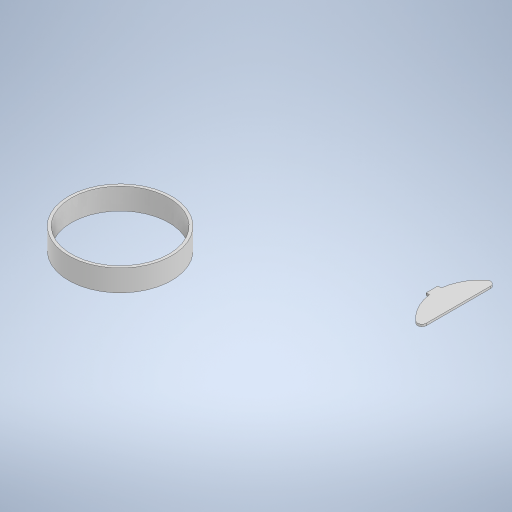
# Autodesk Inventor part: Socle test mesure
Saved by Autodesk Inventor 2024 (Build 280153000, 153)
## iProperties
Created: 2025-01-19
Part Number: Socle test mesure
Material: Générique
Document SubType Name: Modeling
Designer: malam
Density: 1 g/cm^3
Appearance: Par défaut
Author: malam
Autodesk Inventor part; units mm, degrees
ref_plane "YZ Plane" through (0, 0, 0) normal (1, 0, 0) x (0, 1, 0)
ref_plane "XZ Plane" through (0, 0, 0) normal (0, 1, 0) x (-1, 0, 0)
ref_plane "XY Plane" through (0, 0, 0) normal (0, 0, 1) x (1, 0, 0)
sketch "Esquisse1" plane through (0, 0, 0) normal (0, 1, 0) x (-1, 0, 0)
  circle A0 centre (0, 0) radius 45.31
  circle A1 centre (0, 0) radius 47.89
  arc A2 (26.876, -173.3076) -> (26.876, -102.0616) centre (-1.124, -137.6846) ccw
  line L0 (26.876, -105.1346) -> (26.876, -170.2346)
  arc A3 (26.876, -176.5363) -> (26.876, -98.8329) centre (-1.124, -137.6846) ccw
  line L1 (26.876, -170.2346) -> (26.876, -176.5363)
  line L2 (26.876, -105.1346) -> (26.876, -98.8329)
  line L3 (19.5, -32.55) -> (1.5, -32.55)
  line L4 (1.5, -32.55) -> (1.5, 32.55)
  line L5 (1.5, 32.55) -> (19.5, 32.55)
  line L6 (19.5, 32.55) -> (19.5, -32.55)
  line L7 (-1.5, -32.55) -> (-19.5, -32.55)
  line L8 (-19.5, -32.55) -> (-19.5, 32.55)
  line L9 (-19.5, 32.55) -> (-1.5, 32.55)
  line L10 (-1.5, 32.55) -> (-1.5, -32.55)
  line L11 (19.5, -32.55) -> (-19.5, 32.55) construction
  line L12 (19.5, 32.55) -> (-19.5, -32.55) construction
  line L13 (19.5, -32.55) -> (19.5, -43.7402)
  line L14 (19.5, 32.55) -> (19.5, 43.7402)
  arc A4 (-204.4871, -152.7477) -> (-204.4871, -70.9493) centre (-223.9871, -111.8485) ccw
  line L15 (-204.4871, -79.2985) -> (-204.4871, -144.3985)
  line L16 (-204.4871, -144.3985) -> (-204.4871, -152.7477)
  line L17 (-204.4871, -79.2985) -> (-204.4871, -70.9493)
  line L18 (-202.4871, -74.2519) -> (-202.4871, -79.2985)
  line L19 (-202.4871, -79.2985) -> (-202.4871, -144.3985)
  line L20 (-202.4871, -144.3985) -> (-202.4871, -149.4451)
  arc A5 (-202.4871, -149.4451) -> (-202.4871, -74.2519) centre (-223.9871, -111.8485) ccw
  point P0 (0, 0)
  point P1 (0, 0)
  dimension "d0" = 90.62
  dimension "d11" = 2.58
  dimension "d14" = 90.62
  dimension "d15" = 2.58
  dimension "d16" = 18
  dimension "d17" = 65.1
  dimension "d18" = 18
  dimension "d19" = 3
  dimension "d20" = 90.62
  dimension "d22" = 2
  constraints: 42 end point, 10 point on circle, 6 centre point, 4 parallel, 4 point on line, 3 vertical, 2 horizontal, 2 perpendicular, 1 midpoint, 3 other
  measures "d0" diameter of A0
  measures "d11" radial gap between concentric circles of A0 A1
  measures "d14" diameter of A2
  measures "d15" radial gap between concentric circles of A2 A3
  measures "d16" distance of L4.end L6.start
  measures "d17" distance of L3.end L4.end
  measures "d18" distance of L8.end L10.start
  measures "d19" distance between parallel lines of L10 L4
  measures "d20" diameter of A4
  measures "d22" radial gap between concentric circles of A4 A5
extrude "Extrusion1" add sketch "Esquisse1" along normal blind 20 contours A0 L14 A1 L13 | A0 L13 A1 L14
extrude "Extrusion2" add sketch "Esquisse1" along normal blind 2 contours A5 L20 L19 L18
fillet "Congé1" radius 4 2 edges at (202.4871, 1, -149.4451) (202.4871, 1, -74.2519)
sketch "Esquisse2" plane through (0, 2, 0) normal (0, 1, 0) x (1, 0, 0)
  arc A0 (204.4871, 152.7477) -> (204.4871, 70.9493) centre (223.9871, 111.8485) ccw projected
  arc A1 (195.8923, 78.8873) -> (202.4871, 81.9315) centre (198.4871, 81.9315) ccw projected
  line L0 (202.4871, 81.9315) -> (202.4871, 141.7655) projected
  arc A2 (202.4871, 141.7655) -> (195.8923, 144.8097) centre (198.4871, 141.7655) ccw projected
  arc A3 (195.8923, 144.8097) -> (195.8923, 78.8873) centre (223.9871, 111.8485) ccw projected
  arc A4 (204.4871, 155.5558) -> (204.4871, 68.1412) centre (223.9871, 111.8485) ccw
  line L1 (204.4871, 152.7477) -> (204.4871, 155.5558)
  line L2 (204.4871, 70.9493) -> (204.4871, 68.1412)
  line L3 (223.9871, 111.8485) -> (161.6746, 111.8485) construction
  line L4 (176.4441, 106.3485) -> (177.9441, 106.3485)
  line L5 (177.9441, 106.3485) -> (177.9441, 117.3485)
  line L6 (177.9441, 117.3485) -> (176.4441, 117.3485)
  line L7 (176.4441, 117.3485) -> (176.4441, 106.3485)
  line L8 (176.4441, 106.3485) -> (177.9441, 117.3485) construction
  line L9 (177.9441, 106.3485) -> (176.4441, 117.3485) construction
  line L10 (177.9441, 117.3485) -> (181.0277, 117.3485)
  line L11 (177.9441, 106.3485) -> (181.0277, 106.3485)
  point P0 (0, 0)
  point P1 (177.1941, 111.8485)
  dimension "d26" = 95.72
  dimension "d27" = 1.5
  dimension "d28" = 11
  constraints: 22 end point, 5 point on circle, 3 parallel, 2 horizontal, 2 midpoint, 2 perpendicular, 2 point on line, 1 centre point, 1 coincident, 1 vertical
  measures "d26" diameter of A4
  measures "d27" distance of L6.end L5.end
  measures "d28" distance of L5.end L4.end
extrude "Extrusion3" add sketch "Esquisse2" against normal blind 2 contours L10 A3 L11 A0 | A0 L11 L5 L10
sketch "Esquisse3" plane through (0, 2, 0) normal (0, 1, 0) x (1, 0, 0)
  arc A0 (195.8923, 78.8873) -> (202.4871, 81.9315) centre (198.4871, 81.9315) ccw projected
  line L0 (202.4871, 81.9315) -> (202.4871, 141.7655) projected
  arc A1 (202.4871, 141.7655) -> (195.8923, 144.8097) centre (198.4871, 141.7655) ccw projected
  arc A2 (195.8923, 144.8097) -> (181.0277, 117.3485) centre (223.9871, 111.8485) ccw projected
  line L1 (181.0277, 117.3485) -> (177.9441, 117.3485) projected
  line L2 (177.9441, 117.3485) -> (177.9441, 106.3485) projected
  line L3 (177.9441, 106.3485) -> (181.0277, 106.3485) projected
  arc A3 (181.0277, 106.3485) -> (195.8923, 78.8873) centre (223.9871, 111.8485) ccw projected
  point P0 (0, 0)
